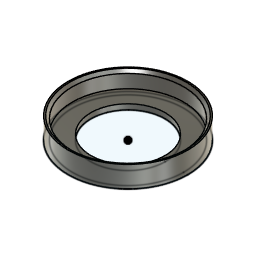
Quick test bearing holder v2 (Autodesk Fusion 360 design; units mm, degrees)
Autodesk Fusion 360 part; units mm, degrees
sketch "Sketch1" plane through (0, 0, 0) normal (0, 0, 1) x (1, 0, 0)
  circle A0 centre (0, 0) radius 22.5
  circle A1 centre (0, 0) radius 20.95
  circle A2 centre (0, 0) radius 14
  dimension "d1" = 45
  dimension "d2" = 41.9
  dimension "d3" = 28
  constraint coincident A0.centre A1.centre
  constraint concentric A1 A2
  measures "d1" diameter of A0
  measures "d2" diameter of A1
  measures "d3" diameter of A2
extrude "Extrude1" add sketch "Sketch1" along normal blind 8 contours A0
extrude "Extrude2" add sketch "Sketch1" along normal blind 2 contours A1
chamfer "Chamfer1" distance 1 angle 45 1 edges at (-19.5323, 7.5758, 8)
